Autodesk Inventor part; units mm, degrees
(part 2 of 3)
  spline S259 degree 2 poles (6.7775, 4.9124) (6.7775, 4.5098) (7.1283, 4.0578) (7.4395, 4.0578) knots 0 0 0 1 2 2 2
  spline S260 degree 2 poles (7.4395, 4.0578) (7.6272, 4.0578) (7.9681, 4.2134) (8.099, 4.3344) knots 0 0 0 1 2 2 2
  line L270 (8.099, 4.3344) -> (8.1212, 4.3344)
  line L271 (8.1212, 4.3344) -> (8.1212, 3.9022)
  spline S261 degree 2 poles (8.1212, 3.9022) (8.0644, 3.875) (7.8915, 3.7984) (7.8223, 3.7811) knots 0 0 0 1 2 2 2
  spline S262 degree 2 poles (7.8223, 3.7811) (7.7235, 3.7515) (7.5679, 3.7218) (7.4469, 3.7218) knots 0 0 0 1 2 2 2
  line L272 (10.2677, 3.7737) -> (9.8823, 3.7737)
  line L273 (9.8823, 3.7737) -> (9.8823, 5.0779)
  spline S263 degree 2 poles (9.8823, 5.0779) (9.8823, 5.236) (9.8527, 5.5077) (9.8082, 5.5892) knots 0 0 0 1 2 2 2
  spline S264 degree 2 poles (9.8082, 5.5892) (9.7613, 5.6756) (9.5933, 5.7596) (9.4501, 5.7596) knots 0 0 0 1 2 2 2
  spline S265 degree 2 poles (9.4501, 5.7596) (9.3068, 5.7596) (9.003, 5.6065) (8.8573, 5.483) knots 0 0 0 1 2 2 2
  line L274 (8.8573, 5.483) -> (8.8573, 3.7737)
  line L275 (8.8573, 3.7737) -> (8.472, 3.7737)
  line L276 (8.472, 3.7737) -> (8.472, 6.9576)
  line L277 (8.472, 6.9576) -> (8.8573, 6.9576)
  line L278 (8.8573, 6.9576) -> (8.8573, 5.8065)
  spline S266 degree 2 poles (8.8573, 5.8065) (9.0302, 5.9621) (9.3636, 6.1252) (9.5514, 6.1252) knots 0 0 0 1 2 2 2
  spline S267 degree 2 poles (9.5514, 6.1252) (9.8873, 6.1252) (10.2677, 5.6806) (10.2677, 5.2582) knots 0 0 0 1 2 2 2
  line L279 (10.2677, 5.2582) -> (10.2677, 3.7737)
  line L280 (14.0221, 4.821) -> (13.659, 4.821)
  line L281 (13.659, 4.821) -> (13.659, 3.7737)
  line L282 (13.659, 3.7737) -> (13.2663, 3.7737)
  line L283 (13.2663, 3.7737) -> (13.2663, 4.821)
  line L284 (13.2663, 4.821) -> (11.9201, 4.821)
  line L285 (11.9201, 4.821) -> (11.9201, 5.2508)
  line L286 (11.9201, 5.2508) -> (13.2836, 6.8217)
  line L287 (13.2836, 6.8217) -> (13.659, 6.8217)
  line L288 (13.659, 6.8217) -> (13.659, 5.1495)
  line L289 (13.659, 5.1495) -> (14.0221, 5.1495)
  line L290 (14.0221, 5.1495) -> (14.0221, 4.821)
  line L291 (13.2663, 5.1495) -> (13.2663, 6.3401)
  line L292 (13.2663, 6.3401) -> (12.2412, 5.1495)
  line L293 (12.2412, 5.1495) -> (13.2663, 5.1495)
  line L294 (16.0747, 3.7737) -> (14.5877, 3.7737)
  line L295 (14.5877, 3.7737) -> (14.5877, 4.0849)
  line L296 (14.5877, 4.0849) -> (15.141, 4.0849)
  line L297 (15.141, 4.0849) -> (15.141, 6.1276)
  line L298 (15.141, 6.1276) -> (14.5877, 6.1276)
  line L299 (14.5877, 6.1276) -> (14.5877, 6.4067)
  spline S268 degree 2 poles (14.5877, 6.4067) (14.9014, 6.4067) (15.1978, 6.5846) (15.2176, 6.8316) knots 0 0 0 1 2 2 2
  line L300 (15.2176, 6.8316) -> (15.5337, 6.8316)
  line L301 (15.5337, 6.8316) -> (15.5337, 4.0849)
  line L302 (15.5337, 4.0849) -> (16.0747, 4.0849)
  line L303 (16.0747, 4.0849) -> (16.0747, 3.7737)
  line L304 (17.2899, 3.7737) -> (16.8009, 3.7737)
  line L305 (16.8009, 3.7737) -> (16.8009, 4.3566)
  line L306 (16.8009, 4.3566) -> (17.2899, 4.3566)
  line L307 (17.2899, 4.3566) -> (17.2899, 3.7737)
  spline S269 degree 2 poles (19.8019, 5.2977) (19.8019, 4.4777) (19.3252, 3.7095) (18.8287, 3.7095) knots 0 0 0 1 2 2 2
  spline S270 degree 2 poles (18.8287, 3.7095) (18.3249, 3.7095) (17.8531, 4.4925) (17.8531, 5.2952) knots 0 0 0 1 2 2 2
  spline S271 degree 2 poles (17.8531, 5.2952) (17.8531, 6.1202) (18.3298, 6.8835) (18.8287, 6.8835) knots 0 0 0 1 2 2 2
  spline S272 degree 2 poles (18.8287, 6.8835) (19.3302, 6.8835) (19.8019, 6.0931) (19.8019, 5.2977) knots 0 0 0 1 2 2 2
  spline S273 degree 2 poles (19.2783, 4.369) (19.3376, 4.5197) (19.387, 4.984) (19.387, 5.2977) knots 0 0 0 1 2 2 2
  spline S274 degree 2 poles (19.387, 5.2977) (19.387, 5.6114) (19.3376, 6.0733) (19.2758, 6.2289) knots 0 0 0 1 2 2 2
  spline S275 degree 2 poles (19.2758, 6.2289) (19.2141, 6.3845) (18.9992, 6.5451) (18.8287, 6.5451) knots 0 0 0 1 2 2 2
  spline S276 degree 2 poles (18.8287, 6.5451) (18.6583, 6.5451) (18.4385, 6.3845) (18.3743, 6.224) knots 0 0 0 1 2 2 2
  spline S277 degree 2 poles (18.3743, 6.224) (18.3125, 6.0684) (18.268, 5.5941) (18.268, 5.2952) knots 0 0 0 1 2 2 2
  spline S278 degree 2 poles (18.268, 5.2952) (18.268, 4.9741) (18.3076, 4.5444) (18.3718, 4.3764) knots 0 0 0 1 2 2 2
  spline S279 degree 2 poles (18.3718, 4.3764) (18.4311, 4.2183) (18.6509, 4.0479) (18.8287, 4.0479) knots 0 0 0 1 2 2 2
  spline S280 degree 2 poles (18.8287, 4.0479) (18.9967, 4.0479) (19.2165, 4.2084) (19.2783, 4.369) knots 0 0 0 1 2 2 2
  spline S281 degree 2 poles (22.0892, 5.2977) (22.0892, 4.4777) (21.6124, 3.7095) (21.116, 3.7095) knots 0 0 0 1 2 2 2
  spline S282 degree 2 poles (21.116, 3.7095) (20.6121, 3.7095) (20.1403, 4.4925) (20.1403, 5.2952) knots 0 0 0 1 2 2 2
  spline S283 degree 2 poles (20.1403, 5.2952) (20.1403, 6.1202) (20.617, 6.8835) (21.116, 6.8835) knots 0 0 0 1 2 2 2
  spline S284 degree 2 poles (21.116, 6.8835) (21.6174, 6.8835) (22.0892, 6.0931) (22.0892, 5.2977) knots 0 0 0 1 2 2 2
  spline S285 degree 2 poles (21.5655, 4.369) (21.6248, 4.5197) (21.6742, 4.984) (21.6742, 5.2977) knots 0 0 0 1 2 2 2
  spline S286 degree 2 poles (21.6742, 5.2977) (21.6742, 5.6114) (21.6248, 6.0733) (21.563, 6.2289) knots 0 0 0 1 2 2 2
  spline S287 degree 2 poles (21.563, 6.2289) (21.5013, 6.3845) (21.2864, 6.5451) (21.116, 6.5451) knots 0 0 0 1 2 2 2
  spline S288 degree 2 poles (21.116, 6.5451) (20.9455, 6.5451) (20.7257, 6.3845) (20.6615, 6.224) knots 0 0 0 1 2 2 2
  spline S289 degree 2 poles (20.6615, 6.224) (20.5997, 6.0684) (20.5553, 5.5941) (20.5553, 5.2952) knots 0 0 0 1 2 2 2
  spline S290 degree 2 poles (20.5553, 5.2952) (20.5553, 4.9741) (20.5948, 4.5444) (20.659, 4.3764) knots 0 0 0 1 2 2 2
  spline S291 degree 2 poles (20.659, 4.3764) (20.7183, 4.2183) (20.9381, 4.0479) (21.116, 4.0479) knots 0 0 0 1 2 2 2
  spline S292 degree 2 poles (21.116, 4.0479) (21.2839, 4.0479) (21.5038, 4.2084) (21.5655, 4.369) knots 0 0 0 1 2 2 2
  spline S293 degree 2 poles (23.3019, 6.5327) (23.1908, 6.5327) (22.971, 6.4784) (22.8647, 6.4364) knots 0 0 0 1 2 2 2
  spline S294 degree 2 poles (22.8647, 6.4364) (22.7659, 6.3944) (22.6202, 6.3055) (22.5634, 6.266) knots 0 0 0 1 2 2 2
  line L308 (22.5634, 6.266) -> (22.5387, 6.266)
  line L309 (22.5387, 6.266) -> (22.5387, 6.6982)
  spline S295 degree 2 poles (22.5387, 6.6982) (22.6721, 6.7698) (23.129, 6.8859) (23.334, 6.8859) knots 0 0 0 1 2 2 2
  spline S296 degree 2 poles (23.334, 6.8859) (23.5415, 6.8859) (23.8503, 6.8019) (23.9763, 6.713) knots 0 0 0 1 2 2 2
  spline S297 degree 2 poles (23.9763, 6.713) (24.1096, 6.6167) (24.248, 6.3376) (24.248, 6.1499) knots 0 0 0 1 2 2 2
  spline S298 degree 2 poles (24.248, 6.1499) (24.248, 5.8979) (23.917, 5.5175) (23.6848, 5.4681) knots 0 0 0 1 2 2 2
  line L310 (23.6848, 5.4681) -> (23.6848, 5.4385)
  spline S299 degree 2 poles (23.6848, 5.4385) (23.7811, 5.4187) (24.001, 5.3298) (24.0948, 5.2409) knots 0 0 0 1 2 2 2
  spline S300 degree 2 poles (24.0948, 5.2409) (24.1887, 5.1544) (24.3072, 4.8778) (24.3072, 4.6777) knots 0 0 0 1 2 2 2
  spline S301 degree 2 poles (24.3072, 4.6777) (24.3072, 4.4727) (24.1664, 4.1245) (24.038, 3.9911) knots 0 0 0 1 2 2 2
  spline S302 degree 2 poles (24.038, 3.9911) (23.9046, 3.8527) (23.5267, 3.7095) (23.2871, 3.7095) knots 0 0 0 1 2 2 2
  spline S303 degree 2 poles (23.2871, 3.7095) (23.0574, 3.7095) (22.6079, 3.8206) (22.4547, 3.8972) knots 0 0 0 1 2 2 2
  line L311 (22.4547, 3.8972) -> (22.4547, 4.3295)
  line L312 (22.4547, 4.3295) -> (22.4844, 4.3295)
  spline S304 degree 2 poles (22.4844, 4.3295) (22.6128, 4.2356) (23.0475, 4.0627) (23.2624, 4.0627) knots 0 0 0 1 2 2 2
  spline S305 degree 2 poles (23.2624, 4.0627) (23.3884, 4.0627) (23.6403, 4.1417) (23.7243, 4.2331) knots 0 0 0 1 2 2 2
  spline S306 degree 2 poles (23.7243, 4.2331) (23.8058, 4.3245) (23.8923, 4.5419) (23.8923, 4.7074) knots 0 0 0 1 2 2 2
  spline S307 degree 2 poles (23.8923, 4.7074) (23.8923, 4.8729) (23.7959, 5.0878) (23.7095, 5.1495) knots 0 0 0 1 2 2 2
  spline S308 degree 2 poles (23.7095, 5.1495) (23.623, 5.2113) (23.3884, 5.2582) (23.2501, 5.2582) knots 0 0 0 1 2 2 2
  line L313 (23.2501, 5.2582) -> (23.0772, 5.2582)
  line L314 (23.0772, 5.2582) -> (23.0772, 5.5966)
  line L315 (23.0772, 5.5966) -> (23.213, 5.5966)
  spline S309 degree 2 poles (23.213, 5.5966) (23.4872, 5.5966) (23.833, 5.8584) (23.833, 6.1079) knots 0 0 0 1 2 2 2
  spline S310 degree 2 poles (23.833, 6.1079) (23.833, 6.224) (23.7441, 6.3895) (23.6724, 6.4389) knots 0 0 0 1 2 2 2
  spline S311 degree 2 poles (23.6724, 6.4389) (23.5959, 6.4907) (23.4081, 6.5327) (23.3019, 6.5327) knots 0 0 0 1 2 2 2
  line L316 (27.9085, 3.7737) -> (27.4367, 3.7737)
  line L317 (27.4367, 3.7737) -> (26.881, 4.6333)
  line L318 (26.881, 4.6333) -> (26.3104, 3.7737)
  line L319 (26.3104, 3.7737) -> (25.8732, 3.7737)
  line L320 (25.8732, 3.7737) -> (26.6661, 4.9074)
  line L321 (26.6661, 4.9074) -> (25.8806, 6.0609)
  line L322 (25.8806, 6.0609) -> (26.3524, 6.0609)
  line L323 (26.3524, 6.0609) -> (26.9057, 5.2088)
  line L324 (26.9057, 5.2088) -> (27.4713, 6.0609)
  line L325 (27.4713, 6.0609) -> (27.9085, 6.0609)
  line L326 (27.9085, 6.0609) -> (27.1206, 4.9321)
  line L327 (27.1206, 4.9321) -> (27.9085, 3.7737)
  spline S312 degree 2 poles (30.2822, 6.5327) (30.1711, 6.5327) (29.9512, 6.4784) (29.845, 6.4364) knots 0 0 0 1 2 2 2
  spline S313 degree 2 poles (29.845, 6.4364) (29.7462, 6.3944) (29.6005, 6.3055) (29.5437, 6.266) knots 0 0 0 1 2 2 2
  line L328 (29.5437, 6.266) -> (29.519, 6.266)
  line L329 (29.519, 6.266) -> (29.519, 6.6982)
  spline S314 degree 2 poles (29.519, 6.6982) (29.6523, 6.7698) (30.1093, 6.8859) (30.3143, 6.8859) knots 0 0 0 1 2 2 2
  spline S315 degree 2 poles (30.3143, 6.8859) (30.5218, 6.8859) (30.8305, 6.8019) (30.9565, 6.713) knots 0 0 0 1 2 2 2
  spline S316 degree 2 poles (30.9565, 6.713) (31.0899, 6.6167) (31.2282, 6.3376) (31.2282, 6.1499) knots 0 0 0 1 2 2 2
  spline S317 degree 2 poles (31.2282, 6.1499) (31.2282, 5.8979) (30.8972, 5.5175) (30.6651, 5.4681) knots 0 0 0 1 2 2 2
  line L330 (30.6651, 5.4681) -> (30.6651, 5.4385)
  spline S318 degree 2 poles (30.6651, 5.4385) (30.7614, 5.4187) (30.9812, 5.3298) (31.0751, 5.2409) knots 0 0 0 1 2 2 2
  spline S319 degree 2 poles (31.0751, 5.2409) (31.1689, 5.1544) (31.2875, 4.8778) (31.2875, 4.6777) knots 0 0 0 1 2 2 2
  spline S320 degree 2 poles (31.2875, 4.6777) (31.2875, 4.4727) (31.1467, 4.1245) (31.0183, 3.9911) knots 0 0 0 1 2 2 2
  spline S321 degree 2 poles (31.0183, 3.9911) (30.8849, 3.8527) (30.507, 3.7095) (30.2674, 3.7095) knots 0 0 0 1 2 2 2
  spline S322 degree 2 poles (30.2674, 3.7095) (30.0377, 3.7095) (29.5881, 3.8206) (29.435, 3.8972) knots 0 0 0 1 2 2 2
  line L331 (29.435, 3.8972) -> (29.435, 4.3295)
  line L332 (29.435, 4.3295) -> (29.4646, 4.3295)
  spline S323 degree 2 poles (29.4646, 4.3295) (29.5931, 4.2356) (30.0278, 4.0627) (30.2427, 4.0627) knots 0 0 0 1 2 2 2
  spline S324 degree 2 poles (30.2427, 4.0627) (30.3687, 4.0627) (30.6206, 4.1417) (30.7046, 4.2331) knots 0 0 0 1 2 2 2
  spline S325 degree 2 poles (30.7046, 4.2331) (30.7861, 4.3245) (30.8725, 4.5419) (30.8725, 4.7074) knots 0 0 0 1 2 2 2
  spline S326 degree 2 poles (30.8725, 4.7074) (30.8725, 4.8729) (30.7762, 5.0878) (30.6898, 5.1495) knots 0 0 0 1 2 2 2
  spline S327 degree 2 poles (30.6898, 5.1495) (30.6033, 5.2113) (30.3687, 5.2582) (30.2303, 5.2582) knots 0 0 0 1 2 2 2
  line L333 (30.2303, 5.2582) -> (30.0574, 5.2582)
  line L334 (30.0574, 5.2582) -> (30.0574, 5.5966)
  line L335 (30.0574, 5.5966) -> (30.1933, 5.5966)
  spline S328 degree 2 poles (30.1933, 5.5966) (30.4675, 5.5966) (30.8133, 5.8584) (30.8133, 6.1079) knots 0 0 0 1 2 2 2
  spline S329 degree 2 poles (30.8133, 6.1079) (30.8133, 6.224) (30.7243, 6.3895) (30.6527, 6.4389) knots 0 0 0 1 2 2 2
  spline S330 degree 2 poles (30.6527, 6.4389) (30.5761, 6.4907) (30.3884, 6.5327) (30.2822, 6.5327) knots 0 0 0 1 2 2 2
  line L336 (33.7081, 4.821) -> (33.345, 4.821)
  line L337 (33.345, 4.821) -> (33.345, 3.7737)
  line L338 (33.345, 3.7737) -> (32.9523, 3.7737)
  line L339 (32.9523, 3.7737) -> (32.9523, 4.821)
  line L340 (32.9523, 4.821) -> (31.6061, 4.821)
  line L341 (31.6061, 4.821) -> (31.6061, 5.2508)
  line L342 (31.6061, 5.2508) -> (32.9696, 6.8217)
  line L343 (32.9696, 6.8217) -> (33.345, 6.8217)
  line L344 (33.345, 6.8217) -> (33.345, 5.1495)
  line L345 (33.345, 5.1495) -> (33.7081, 5.1495)
  line L346 (33.7081, 5.1495) -> (33.7081, 4.821)
  line L347 (32.9523, 5.1495) -> (32.9523, 6.3401)
  line L348 (32.9523, 6.3401) -> (31.9272, 5.1495)
  line L349 (31.9272, 5.1495) -> (32.9523, 5.1495)
  line L350 (34.6887, 3.7737) -> (34.1996, 3.7737)
  line L351 (34.1996, 3.7737) -> (34.1996, 4.3566)
  line L352 (34.1996, 4.3566) -> (34.6887, 4.3566)
  line L353 (34.6887, 4.3566) -> (34.6887, 3.7737)
  spline S331 degree 2 poles (36.1263, 6.5327) (36.0151, 6.5327) (35.7953, 6.4784) (35.6891, 6.4364) knots 0 0 0 1 2 2 2
  spline S332 degree 2 poles (35.6891, 6.4364) (35.5903, 6.3944) (35.4445, 6.3055) (35.3877, 6.266) knots 0 0 0 1 2 2 2
  line L354 (35.3877, 6.266) -> (35.363, 6.266)
  line L355 (35.363, 6.266) -> (35.363, 6.6982)
  spline S333 degree 2 poles (35.363, 6.6982) (35.4964, 6.7698) (35.9534, 6.8859) (36.1584, 6.8859) knots 0 0 0 1 2 2 2
  spline S334 degree 2 poles (36.1584, 6.8859) (36.3659, 6.8859) (36.6746, 6.8019) (36.8006, 6.713) knots 0 0 0 1 2 2 2
  spline S335 degree 2 poles (36.8006, 6.713) (36.934, 6.6167) (37.0723, 6.3376) (37.0723, 6.1499) knots 0 0 0 1 2 2 2
  spline S336 degree 2 poles (37.0723, 6.1499) (37.0723, 5.8979) (36.7413, 5.5175) (36.5091, 5.4681) knots 0 0 0 1 2 2 2
  line L356 (36.5091, 5.4681) -> (36.5091, 5.4385)
  spline S337 degree 2 poles (36.5091, 5.4385) (36.6054, 5.4187) (36.8253, 5.3298) (36.9191, 5.2409) knots 0 0 0 1 2 2 2
  spline S338 degree 2 poles (36.9191, 5.2409) (37.013, 5.1544) (37.1316, 4.8778) (37.1316, 4.6777) knots 0 0 0 1 2 2 2
  spline S339 degree 2 poles (37.1316, 4.6777) (37.1316, 4.4727) (36.9908, 4.1245) (36.8623, 3.9911) knots 0 0 0 1 2 2 2
  spline S340 degree 2 poles (36.8623, 3.9911) (36.7289, 3.8527) (36.351, 3.7095) (36.1114, 3.7095) knots 0 0 0 1 2 2 2
  spline S341 degree 2 poles (36.1114, 3.7095) (35.8817, 3.7095) (35.4322, 3.8206) (35.279, 3.8972) knots 0 0 0 1 2 2 2
  line L357 (35.279, 3.8972) -> (35.279, 4.3295)
  line L358 (35.279, 4.3295) -> (35.3087, 4.3295)
  spline S342 degree 2 poles (35.3087, 4.3295) (35.4371, 4.2356) (35.8719, 4.0627) (36.0867, 4.0627) knots 0 0 0 1 2 2 2
  spline S343 degree 2 poles (36.0867, 4.0627) (36.2127, 4.0627) (36.4647, 4.1417) (36.5486, 4.2331) knots 0 0 0 1 2 2 2
  spline S344 degree 2 poles (36.5486, 4.2331) (36.6301, 4.3245) (36.7166, 4.5419) (36.7166, 4.7074) knots 0 0 0 1 2 2 2
  spline S345 degree 2 poles (36.7166, 4.7074) (36.7166, 4.8729) (36.6203, 5.0878) (36.5338, 5.1495) knots 0 0 0 1 2 2 2
  spline S346 degree 2 poles (36.5338, 5.1495) (36.4474, 5.2113) (36.2127, 5.2582) (36.0744, 5.2582) knots 0 0 0 1 2 2 2
  line L359 (36.0744, 5.2582) -> (35.9015, 5.2582)
  line L360 (35.9015, 5.2582) -> (35.9015, 5.5966)
  line L361 (35.9015, 5.5966) -> (36.0373, 5.5966)
  spline S347 degree 2 poles (36.0373, 5.5966) (36.3115, 5.5966) (36.6573, 5.8584) (36.6573, 6.1079) knots 0 0 0 1 2 2 2
  spline S348 degree 2 poles (36.6573, 6.1079) (36.6573, 6.224) (36.5684, 6.3895) (36.4968, 6.4389) knots 0 0 0 1 2 2 2
  spline S349 degree 2 poles (36.4968, 6.4389) (36.4202, 6.4907) (36.2325, 6.5327) (36.1263, 6.5327) knots 0 0 0 1 2 2 2
  spline S350 degree 2 poles (39.4386, 4.742) (39.4386, 4.5221) (39.2978, 4.1467) (39.1693, 4.0084) knots 0 0 0 1 2 2 2
  spline S351 degree 2 poles (39.1693, 4.0084) (39.0409, 3.87) (38.658, 3.7095) (38.4209, 3.7095) knots 0 0 0 1 2 2 2
  spline S352 degree 2 poles (38.4209, 3.7095) (38.2035, 3.7095) (37.7787, 3.8058) (37.6231, 3.8824) knots 0 0 0 1 2 2 2
  line L362 (37.6231, 3.8824) -> (37.6231, 4.3146)
  line L363 (37.6231, 4.3146) -> (37.6527, 4.3146)
  spline S353 degree 2 poles (37.6527, 4.3146) (37.6997, 4.2801) (37.875, 4.1911) (37.9812, 4.1516) knots 0 0 0 1 2 2 2
  spline S354 degree 2 poles (37.9812, 4.1516) (38.1023, 4.1096) (38.3023, 4.0627) (38.4283, 4.0627) knots 0 0 0 1 2 2 2
  spline S355 degree 2 poles (38.4283, 4.0627) (38.5518, 4.0627) (38.784, 4.1516) (38.868, 4.248) knots 0 0 0 1 2 2 2
  spline S356 degree 2 poles (38.868, 4.248) (38.9446, 4.3393) (39.0236, 4.5814) (39.0236, 4.7444) knots 0 0 0 1 2 2 2
  spline S357 degree 2 poles (39.0236, 4.7444) (39.0236, 4.9074) (38.9347, 5.1149) (38.8507, 5.1841) knots 0 0 0 1 2 2 2
  spline S358 degree 2 poles (38.8507, 5.1841) (38.7642, 5.2607) (38.5074, 5.3249) (38.3517, 5.3249) knots 0 0 0 1 2 2 2
  spline S359 degree 2 poles (38.3517, 5.3249) (38.1838, 5.3249) (37.8503, 5.273) (37.7491, 5.2508) knots 0 0 0 1 2 2 2
  line L364 (37.7491, 5.2508) -> (37.7491, 6.8217)
  line L365 (37.7491, 6.8217) -> (39.4213, 6.8217)
  line L366 (39.4213, 6.8217) -> (39.4213, 6.4636)
  line L367 (39.4213, 6.4636) -> (38.1418, 6.4636)
  line L368 (38.1418, 6.4636) -> (38.1418, 5.6509)
  spline S360 degree 2 poles (38.1418, 5.6509) (38.2159, 5.6608) (38.3592, 5.6682) (38.4184, 5.6682) knots 0 0 0 1 2 2 2
  spline S361 degree 2 poles (38.4184, 5.6682) (38.6531, 5.6682) (38.9767, 5.5916) (39.1249, 5.478) knots 0 0 0 1 2 2 2
  spline S362 degree 2 poles (39.1249, 5.478) (39.2755, 5.3644) (39.4386, 5.0186) (39.4386, 4.742) knots 0 0 0 1 2 2 2
  spline S363 degree 2 poles (39.7942, 5.8312) (39.7942, 6.0659) (39.9474, 6.4561) (40.0808, 6.5969) knots 0 0 0 1 2 2 2
  spline S364 degree 2 poles (40.0808, 6.5969) (40.2067, 6.7328) (40.5748, 6.8835) (40.7625, 6.8835) knots 0 0 0 1 2 2 2
  spline S365 degree 2 poles (40.7625, 6.8835) (40.9724, 6.8835) (41.3133, 6.7427) (41.4393, 6.6093) knots 0 0 0 1 2 2 2
  spline S366 degree 2 poles (41.4393, 6.6093) (41.5973, 6.4413) (41.7702, 5.8979) (41.7702, 5.4805) knots 0 0 0 1 2 2 2
  spline S367 degree 2 poles (41.7702, 5.4805) (41.7702, 5.1026) (41.5998, 4.4258) (41.4343, 4.201) knots 0 0 0 1 2 2 2
  spline S368 degree 2 poles (41.4343, 4.201) (41.259, 3.9639) (40.765, 3.7144) (40.4043, 3.7144) knots 0 0 0 1 2 2 2
  spline S369 degree 2 poles (40.4043, 3.7144) (40.3228, 3.7144) (40.1376, 3.7317) (40.0585, 3.7564) knots 0 0 0 1 2 2 2
  line L369 (40.0585, 3.7564) -> (40.0585, 4.1492)
  line L370 (40.0585, 4.1492) -> (40.0783, 4.1492)
  spline S370 degree 2 poles (40.0783, 4.1492) (40.1302, 4.1195) (40.3475, 4.0676) (40.4587, 4.0676) knots 0 0 0 1 2 2 2
  spline S371 degree 2 poles (40.4587, 4.0676) (40.8588, 4.0676) (41.3158, 4.5962) (41.3479, 5.0853) knots 0 0 0 1 2 2 2
  spline S372 degree 2 poles (41.3479, 5.0853) (41.1849, 4.9741) (40.8885, 4.8729) (40.7131, 4.8729) knots 0 0 0 1 2 2 2
  spline S373 degree 2 poles (40.7131, 4.8729) (40.5451, 4.8729) (40.266, 4.947) (40.1252, 5.0532) knots 0 0 0 1 2 2 2
  spline S374 degree 2 poles (40.1252, 5.0532) (39.9622, 5.1791) (39.7942, 5.562) (39.7942, 5.8312) knots 0 0 0 1 2 2 2
  spline S375 degree 2 poles (41.3578, 5.5719) (41.3578, 5.8806) (41.2441, 6.2709) (41.1429, 6.3771) knots 0 0 0 1 2 2 2
  spline S376 degree 2 poles (41.1429, 6.3771) (41.0539, 6.4759) (40.8687, 6.55) (40.76, 6.55) knots 0 0 0 1 2 2 2
  spline S377 degree 2 poles (40.76, 6.55) (40.5081, 6.55) (40.2092, 6.1894) (40.2092, 5.8485) knots 0 0 0 1 2 2 2
  spline S378 degree 2 poles (40.2092, 5.8485) (40.2092, 5.6559) (40.308, 5.4064) (40.4167, 5.3175) knots 0 0 0 1 2 2 2
  spline S379 degree 2 poles (40.4167, 5.3175) (40.4957, 5.2532) (40.6909, 5.2113) (40.8045, 5.2113) knots 0 0 0 1 2 2 2
  spline S380 degree 2 poles (40.8045, 5.2113) (40.9354, 5.2113) (41.2367, 5.3026) (41.3503, 5.3792) knots 0 0 0 1 2 2 2
  spline S381 degree 2 poles (41.3503, 5.3792) (41.3528, 5.4089) (41.3578, 5.5101) (41.3578, 5.5719) knots 0 0 0 1 2 2 2
  spline S382 degree 2 poles (45.4111, 4.9173) (45.4111, 4.3393) (44.8553, 3.7095) (44.3909, 3.7095) knots 0 0 0 1 2 2 2
  spline S383 degree 2 poles (44.3909, 3.7095) (43.9142, 3.7095) (43.3684, 4.3591) (43.3684, 4.9173) knots 0 0 0 1 2 2 2
  spline S384 degree 2 poles (43.3684, 4.9173) (43.3684, 5.4904) (43.9315, 6.1252) (44.3909, 6.1252) knots 0 0 0 1 2 2 2
  spline S385 degree 2 poles (44.3909, 6.1252) (44.8553, 6.1252) (45.4111, 5.4928) (45.4111, 4.9173) knots 0 0 0 1 2 2 2
  spline S386 degree 2 poles (45.0134, 4.9173) (45.0134, 5.3619) (44.6898, 5.7942) (44.3909, 5.7942) knots 0 0 0 1 2 2 2
  spline S387 degree 2 poles (44.3909, 5.7942) (44.0921, 5.7942) (43.766, 5.3619) (43.766, 4.9173) knots 0 0 0 1 2 2 2
  spline S388 degree 2 poles (43.766, 4.9173) (43.766, 4.4851) (44.0921, 4.0405) (44.3909, 4.0405) knots 0 0 0 1 2 2 2
  spline S389 degree 2 poles (44.3909, 4.0405) (44.6873, 4.0405) (45.0134, 4.4777) (45.0134, 4.9173) knots 0 0 0 1 2 2 2
  line L371 (47.0092, 6.5871) -> (46.9894, 6.5871)
  spline S390 degree 2 poles (46.9894, 6.5871) (46.9375, 6.6068) (46.7449, 6.6414) (46.6683, 6.6414) knots 0 0 0 1 2 2 2
  spline S391 degree 2 poles (46.6683, 6.6414) (46.4262, 6.6414) (46.2187, 6.424) (46.2187, 6.1375) knots 0 0 0 1 2 2 2
  line L372 (46.2187, 6.1375) -> (46.2187, 6.0609)
  line L373 (46.2187, 6.0609) -> (46.856, 6.0609)
  line L374 (46.856, 6.0609) -> (46.856, 5.7423)
  line L375 (46.856, 5.7423) -> (46.2311, 5.7423)
  line L376 (46.2311, 5.7423) -> (46.2311, 3.7737)
  line L377 (46.2311, 3.7737) -> (45.8458, 3.7737)
  line L378 (45.8458, 3.7737) -> (45.8458, 5.7423)
  line L379 (45.8458, 5.7423) -> (45.5864, 5.7423)
  line L380 (45.5864, 5.7423) -> (45.5864, 6.0609)
  line L381 (45.5864, 6.0609) -> (45.8458, 6.0609)
  line L382 (45.8458, 6.0609) -> (45.8458, 6.1375)
  spline S392 degree 2 poles (45.8458, 6.1375) (45.8458, 6.5475) (46.2434, 6.9773) (46.614, 6.9773) knots 0 0 0 1 2 2 2
  spline S393 degree 2 poles (46.614, 6.9773) (46.7202, 6.9773) (46.9252, 6.9551) (47.0092, 6.9403) knots 0 0 0 1 2 2 2
  line L383 (47.0092, 6.9403) -> (47.0092, 6.5871)
  line L384 (48.343, 6.5871) -> (48.3232, 6.5871)
  spline S394 degree 2 poles (48.3232, 6.5871) (48.2713, 6.6068) (48.0787, 6.6414) (48.0021, 6.6414) knots 0 0 0 1 2 2 2
  spline S395 degree 2 poles (48.0021, 6.6414) (47.76, 6.6414) (47.5526, 6.424) (47.5526, 6.1375) knots 0 0 0 1 2 2 2
  line L385 (47.5526, 6.1375) -> (47.5526, 6.0609)
  line L386 (47.5526, 6.0609) -> (48.1898, 6.0609)
  line L387 (48.1898, 6.0609) -> (48.1898, 5.7423)
  line L388 (48.1898, 5.7423) -> (47.5649, 5.7423)
  line L389 (47.5649, 5.7423) -> (47.5649, 3.7737)
  line L390 (47.5649, 3.7737) -> (47.1796, 3.7737)
  line L391 (47.1796, 3.7737) -> (47.1796, 5.7423)
  line L392 (47.1796, 5.7423) -> (46.9202, 5.7423)
  line L393 (46.9202, 5.7423) -> (46.9202, 6.0609)
  line L394 (46.9202, 6.0609) -> (47.1796, 6.0609)
  line L395 (47.1796, 6.0609) -> (47.1796, 6.1375)
  spline S396 degree 2 poles (47.1796, 6.1375) (47.1796, 6.5475) (47.5773, 6.9773) (47.9478, 6.9773) knots 0 0 0 1 2 2 2
  spline S397 degree 2 poles (47.9478, 6.9773) (48.054, 6.9773) (48.259, 6.9551) (48.343, 6.9403) knots 0 0 0 1 2 2 2
  line L396 (48.343, 6.9403) -> (48.343, 6.5871)
  spline S398 degree 2 poles (49.0914, 3.7194) (48.8617, 3.7194) (48.464, 3.8429) (48.3331, 3.912) knots 0 0 0 1 2 2 2
  line L397 (48.3331, 3.912) -> (48.3331, 4.3443)
  line L398 (48.3331, 4.3443) -> (48.3528, 4.3443)
  spline S399 degree 2 poles (48.3528, 4.3443) (48.4022, 4.3048) (48.5356, 4.2109) (48.6468, 4.159) knots 0 0 0 1 2 2 2
  spline S400 degree 2 poles (48.6468, 4.159) (48.7431, 4.1121) (48.9802, 4.0429) (49.1062, 4.0429) knots 0 0 0 1 2 2 2
  spline S401 degree 2 poles (49.1062, 4.0429) (49.1976, 4.0429) (49.4075, 4.0849) (49.4569, 4.1195) knots 0 0 0 1 2 2 2
  spline S402 degree 2 poles (49.4569, 4.1195) (49.5286, 4.1664) (49.5928, 4.2727) (49.5928, 4.3813) knots 0 0 0 1 2 2 2
  spline S403 degree 2 poles (49.5928, 4.3813) (49.5928, 4.5172) (49.4446, 4.658) (49.2544, 4.7049) knots 0 0 0 1 2 2 2
  spline S404 degree 2 poles (49.2544, 4.7049) (49.1803, 4.7222) (48.9432, 4.7716) (48.8419, 4.7988) knots 0 0 0 1 2 2 2
  spline S405 degree 2 poles (48.8419, 4.7988) (48.5801, 4.8753) (48.343, 5.1915) (48.343, 5.4163) knots 0 0 0 1 2 2 2
  spline S406 degree 2 poles (48.343, 5.4163) (48.343, 5.7275) (48.8098, 6.1153) (49.1951, 6.1153) knots 0 0 0 1 2 2 2
  spline S407 degree 2 poles (49.1951, 6.1153) (49.3853, 6.1153) (49.7706, 6.0214) (49.9015, 5.9498) knots 0 0 0 1 2 2 2
  line L399 (49.9015, 5.9498) -> (49.9015, 5.5373)
  line L400 (49.9015, 5.5373) -> (49.8818, 5.5373)
  spline S408 degree 2 poles (49.8818, 5.5373) (49.7336, 5.6559) (49.373, 5.7917) (49.1877, 5.7917) knots 0 0 0 1 2 2 2
  spline S409 degree 2 poles (49.1877, 5.7917) (48.9975, 5.7917) (48.7357, 5.6312) (48.7357, 5.4706) knots 0 0 0 1 2 2 2
  spline S410 degree 2 poles (48.7357, 5.4706) (48.7357, 5.3249) (48.8913, 5.1841) (49.0642, 5.1396) knots 0 0 0 1 2 2 2
  spline S411 degree 2 poles (49.0642, 5.1396) (49.1482, 5.1174) (49.3606, 5.0729) (49.4767, 5.0458) knots 0 0 0 1 2 2 2
  spline S412 degree 2 poles (49.4767, 5.0458) (49.7286, 4.9815) (49.9855, 4.6876) (49.9855, 4.4332) knots 0 0 0 1 2 2 2
  spline S413 degree 2 poles (49.9855, 4.4332) (49.9855, 4.285) (49.8694, 4.0232) (49.7558, 3.9269) knots 0 0 0 1 2 2 2
  spline S414 degree 2 poles (49.7558, 3.9269) (49.6348, 3.8256) (49.326, 3.7194) (49.0914, 3.7194) knots 0 0 0 1 2 2 2
  spline S415 degree 2 poles (51.3366, 3.7218) (50.7883, 3.7218) (50.1856, 4.3369) (50.1856, 4.905) knots 0 0 0 1 2 2 2
  spline S416 degree 2 poles (50.1856, 4.905) (50.1856, 5.4632) (50.771, 6.1252) (51.2428, 6.1252) knots 0 0 0 1 2 2 2
  spline S417 degree 2 poles (51.2428, 6.1252) (51.4552, 6.1252) (51.7837, 6.0017) (51.9047, 5.8708) knots 0 0 0 1 2 2 2
  spline S418 degree 2 poles (51.9047, 5.8708) (52.0282, 5.7398) (52.1591, 5.3619) (52.1591, 5.0878) knots 0 0 0 1 2 2 2
  line L401 (52.1591, 5.0878) -> (52.1591, 4.8778)
  line L402 (52.1591, 4.8778) -> (50.5759, 4.8778)
  spline S419 degree 2 poles (50.5759, 4.8778) (50.5759, 4.4801) (50.976, 4.0578) (51.3317, 4.0578) knots 0 0 0 1 2 2 2
  spline S420 degree 2 poles (51.3317, 4.0578) (51.4577, 4.0578) (51.7022, 4.1146) (51.801, 4.159) knots 0 0 0 1 2 2 2
  spline S421 degree 2 poles (51.801, 4.159) (51.9047, 4.2084) (52.048, 4.2949) (52.0949, 4.3344) knots 0 0 0 1 2 2 2
  line L403 (52.0949, 4.3344) -> (52.1171, 4.3344)
  line L404 (52.1171, 4.3344) -> (52.1171, 3.9145)
  spline S422 degree 2 poles (52.1171, 3.9145) (52.0505, 3.8873) (51.8479, 3.8083) (51.7689, 3.7861) knots 0 0 0 1 2 2 2
  spline S423 degree 2 poles (51.7689, 3.7861) (51.6577, 3.7539) (51.4749, 3.7218) (51.3366, 3.7218) knots 0 0 0 1 2 2 2
  spline S424 degree 2 poles (51.7837, 5.1717) (51.7788, 5.3273) (51.7145, 5.5546) (51.6528, 5.6312) knots 0 0 0 1 2 2 2
  spline S425 degree 2 poles (51.6528, 5.6312) (51.5861, 5.7176) (51.3761, 5.809) (51.2205, 5.809) knots 0 0 0 1 2 2 2
  spline S426 degree 2 poles (51.2205, 5.809) (51.0674, 5.809) (50.8525, 5.7176) (50.7636, 5.6287) knots 0 0 0 1 2 2 2
  spline S427 degree 2 poles (50.7636, 5.6287) (50.6771, 5.5373) (50.5882, 5.3175) (50.5759, 5.1717) knots 0 0 0 1 2 2 2
  line L405 (50.5759, 5.1717) -> (51.7837, 5.1717)
  spline S428 degree 2 poles (53.241, 3.7292) (52.9273, 3.7292) (52.5741, 4.0874) (52.5741, 4.4752) knots 0 0 0 1 2 2 2
  line L406 (52.5741, 4.4752) -> (52.5741, 5.7423)
  line L407 (52.5741, 5.7423) -> (52.3147, 5.7423)
  line L408 (52.3147, 5.7423) -> (52.3147, 6.0609)
  line L409 (52.3147, 6.0609) -> (52.5741, 6.0609)
  line L410 (52.5741, 6.0609) -> (52.5741, 6.718)
  line L411 (52.5741, 6.718) -> (52.9594, 6.718)
  line L412 (52.9594, 6.718) -> (52.9594, 6.0609)
  line L413 (52.9594, 6.0609) -> (53.6683, 6.0609)
  line L414 (53.6683, 6.0609) -> (53.6683, 5.7423)
  line L415 (53.6683, 5.7423) -> (52.9594, 5.7423)
  line L416 (52.9594, 5.7423) -> (52.9594, 4.653)
  spline S429 degree 2 poles (52.9594, 4.653) (52.9594, 4.4801) (52.9718, 4.2899) (53.0138, 4.2084) knots 0 0 0 1 2 2 2
  spline S430 degree 2 poles (53.0138, 4.2084) (53.0483, 4.1368) (53.204, 4.0652) (53.3373, 4.0652) knots 0 0 0 1 2 2 2
  spline S431 degree 2 poles (53.3373, 4.0652) (53.4312, 4.0652) (53.6066, 4.122) (53.6461, 4.1393) knots 0 0 0 1 2 2 2
  line L417 (53.6461, 4.1393) -> (53.6683, 4.1393)
  line L418 (53.6683, 4.1393) -> (53.6683, 3.7935)
  spline S432 degree 2 poles (53.6683, 3.7935) (53.5596, 3.7638) (53.3373, 3.7292) (53.241, 3.7292) knots 0 0 0 1 2 2 2
  line L419 (57.0844, 3.7737) -> (55.2047, 3.7737)
  line L420 (55.2047, 3.7737) -> (55.2047, 4.206)
  spline S433 degree 2 poles (55.2047, 4.206) (55.4072, 4.3962) (55.7678, 4.7494) (55.9407, 4.9396) knots 0 0 0 1 2 2 2
  spline S434 degree 2 poles (55.9407, 4.9396) (56.289, 5.3224) (56.5434, 5.7818) (56.5434, 6.0264) knots 0 0 0 1 2 2 2
  spline S435 degree 2 poles (56.5434, 6.0264) (56.5434, 6.1548) (56.4644, 6.3475) (56.3927, 6.4092) knots 0 0 0 1 2 2 2
  spline S436 degree 2 poles (56.3927, 6.4092) (56.3211, 6.471) (56.1334, 6.5327) (56.0198, 6.5327) knots 0 0 0 1 2 2 2
  spline S437 degree 2 poles (56.0198, 6.5327) (55.9111, 6.5327) (55.6888, 6.4784) (55.5875, 6.4364) knots 0 0 0 1 2 2 2
  spline S438 degree 2 poles (55.5875, 6.4364) (55.5011, 6.4018) (55.3405, 6.303) (55.2911, 6.2684) knots 0 0 0 1 2 2 2
  line L421 (55.2911, 6.2684) -> (55.2689, 6.2684)
  line L422 (55.2689, 6.2684) -> (55.2689, 6.7031)
  spline S439 degree 2 poles (55.2689, 6.7031) (55.3949, 6.7649) (55.8469, 6.8859) (56.0494, 6.8859) knots 0 0 0 1 2 2 2
  spline S440 degree 2 poles (56.0494, 6.8859) (56.4767, 6.8859) (56.9584, 6.4339) (56.9584, 6.0486) knots 0 0 0 1 2 2 2
  spline S441 degree 2 poles (56.9584, 6.0486) (56.9584, 5.8683) (56.8744, 5.5669) (56.8003, 5.4385) knots 0 0 0 1 2 2 2
  spline S442 degree 2 poles (56.8003, 5.4385) (56.7262, 5.3051) (56.5113, 5.0433) (56.3927, 4.9173) knots 0 0 0 1 2 2 2
  spline S443 degree 2 poles (56.3927, 4.9173) (56.2001, 4.7074) (55.7283, 4.2578) (55.5875, 4.1269) knots 0 0 0 1 2 2 2
  line L423 (55.5875, 4.1269) -> (57.0844, 4.1269)
  line L424 (57.0844, 4.1269) -> (57.0844, 3.7737)
  line L425 (58.1465, 3.7737) -> (57.6574, 3.7737)
  line L426 (57.6574, 3.7737) -> (57.6574, 4.3566)
  line L427 (57.6574, 4.3566) -> (58.1465, 4.3566)
  line L428 (58.1465, 4.3566) -> (58.1465, 3.7737)
  line L429 (60.6758, 6.3648) -> (59.3568, 3.7737)
  line L430 (59.3568, 3.7737) -> (58.922, 3.7737)
  line L431 (58.922, 3.7737) -> (60.3151, 6.4636)
  line L432 (60.3151, 6.4636) -> (58.7417, 6.4636)
  line L433 (58.7417, 6.4636) -> (58.7417, 6.8217)
  line L434 (58.7417, 6.8217) -> (60.6758, 6.8217)
  line L435 (60.6758, 6.8217) -> (60.6758, 6.3648)
  spline S444 degree 2 poles (62.8963, 4.742) (62.8963, 4.5221) (62.7555, 4.1467) (62.6271, 4.0084) knots 0 0 0 1 2 2 2
  spline S445 degree 2 poles (62.6271, 4.0084) (62.4986, 3.87) (62.1158, 3.7095) (61.8787, 3.7095) knots 0 0 0 1 2 2 2
  spline S446 degree 2 poles (61.8787, 3.7095) (61.6613, 3.7095) (61.2364, 3.8058) (61.0808, 3.8824) knots 0 0 0 1 2 2 2
  line L436 (61.0808, 3.8824) -> (61.0808, 4.3146)
  line L437 (61.0808, 4.3146) -> (61.1105, 4.3146)
  spline S447 degree 2 poles (61.1105, 4.3146) (61.1574, 4.2801) (61.3328, 4.1911) (61.439, 4.1516) knots 0 0 0 1 2 2 2
  spline S448 degree 2 poles (61.439, 4.1516) (61.56, 4.1096) (61.7601, 4.0627) (61.8861, 4.0627) knots 0 0 0 1 2 2 2
  spline S449 degree 2 poles (61.8861, 4.0627) (62.0096, 4.0627) (62.2417, 4.1516) (62.3257, 4.248) knots 0 0 0 1 2 2 2
  spline S450 degree 2 poles (62.3257, 4.248) (62.4023, 4.3393) (62.4813, 4.5814) (62.4813, 4.7444) knots 0 0 0 1 2 2 2
  spline S451 degree 2 poles (62.4813, 4.7444) (62.4813, 4.9074) (62.3924, 5.1149) (62.3084, 5.1841) knots 0 0 0 1 2 2 2
  spline S452 degree 2 poles (62.3084, 5.1841) (62.222, 5.2607) (61.9651, 5.3249) (61.8095, 5.3249) knots 0 0 0 1 2 2 2
  spline S453 degree 2 poles (61.8095, 5.3249) (61.6415, 5.3249) (61.3081, 5.273) (61.2068, 5.2508) knots 0 0 0 1 2 2 2
  line L438 (61.2068, 5.2508) -> (61.2068, 6.8217)
  line L439 (61.2068, 6.8217) -> (62.879, 6.8217)
  line L440 (62.879, 6.8217) -> (62.879, 6.4636)
  line L441 (62.879, 6.4636) -> (61.5995, 6.4636)
  line L442 (61.5995, 6.4636) -> (61.5995, 5.6509)
  spline S454 degree 2 poles (61.5995, 5.6509) (61.6736, 5.6608) (61.8169, 5.6682) (61.8762, 5.6682) knots 0 0 0 1 2 2 2
  spline S455 degree 2 poles (61.8762, 5.6682) (62.1108, 5.6682) (62.4344, 5.5916) (62.5826, 5.478) knots 0 0 0 1 2 2 2
  spline S456 degree 2 poles (62.5826, 5.478) (62.7333, 5.3644) (62.8963, 5.0186) (62.8963, 4.742) knots 0 0 0 1 2 2 2
  spline S457 degree 2 poles (65.2329, 5.2977) (65.2329, 4.4777) (64.7562, 3.7095) (64.2597, 3.7095) knots 0 0 0 1 2 2 2
  spline S458 degree 2 poles (64.2597, 3.7095) (63.7559, 3.7095) (63.2841, 4.4925) (63.2841, 5.2952) knots 0 0 0 1 2 2 2
  spline S459 degree 2 poles (63.2841, 5.2952) (63.2841, 6.1202) (63.7608, 6.8835) (64.2597, 6.8835) knots 0 0 0 1 2 2 2
  spline S460 degree 2 poles (64.2597, 6.8835) (64.7612, 6.8835) (65.2329, 6.0931) (65.2329, 5.2977) knots 0 0 0 1 2 2 2
  spline S461 degree 2 poles (64.7093, 4.369) (64.7686, 4.5197) (64.818, 4.984) (64.818, 5.2977) knots 0 0 0 1 2 2 2
  spline S462 degree 2 poles (64.818, 5.2977) (64.818, 5.6114) (64.7686, 6.0733) (64.7068, 6.2289) knots 0 0 0 1 2 2 2
  spline S463 degree 2 poles (64.7068, 6.2289) (64.6451, 6.3845) (64.4302, 6.5451) (64.2597, 6.5451) knots 0 0 0 1 2 2 2
  spline S464 degree 2 poles (64.2597, 6.5451) (64.0893, 6.5451) (63.8695, 6.3845) (63.8053, 6.224) knots 0 0 0 1 2 2 2
  spline S465 degree 2 poles (63.8053, 6.224) (63.7435, 6.0684) (63.6991, 5.5941) (63.6991, 5.2952) knots 0 0 0 1 2 2 2
  spline S466 degree 2 poles (63.6991, 5.2952) (63.6991, 4.9741) (63.7386, 4.5444) (63.8028, 4.3764) knots 0 0 0 1 2 2 2
  spline S467 degree 2 poles (63.8028, 4.3764) (63.8621, 4.2183) (64.0819, 4.0479) (64.2597, 4.0479) knots 0 0 0 1 2 2 2
  spline S468 degree 2 poles (64.2597, 4.0479) (64.4277, 4.0479) (64.6475, 4.2084) (64.7093, 4.369) knots 0 0 0 1 2 2 2
  line L443 (68.7651, 3.7737) -> (68.2933, 3.7737)
  line L444 (68.2933, 3.7737) -> (67.7375, 4.6333)
  line L445 (67.7375, 4.6333) -> (67.167, 3.7737)
  line L446 (67.167, 3.7737) -> (66.7298, 3.7737)
  line L447 (66.7298, 3.7737) -> (67.5226, 4.9074)
  line L448 (67.5226, 4.9074) -> (66.7372, 6.0609)
  line L449 (66.7372, 6.0609) -> (67.2089, 6.0609)
  line L450 (67.2089, 6.0609) -> (67.7622, 5.2088)
  line L451 (67.7622, 5.2088) -> (68.3279, 6.0609)
  line L452 (68.3279, 6.0609) -> (68.7651, 6.0609)
  line L453 (68.7651, 6.0609) -> (67.9771, 4.9321)
  line L454 (67.9771, 4.9321) -> (68.7651, 3.7737)
  spline S469 degree 2 poles (72.2428, 4.7617) (72.2428, 4.5271) (72.0872, 4.1294) (71.9563, 3.996) knots 0 0 0 1 2 2 2
  spline S470 degree 2 poles (71.9563, 3.996) (71.8205, 3.8552) (71.4796, 3.7095) (71.2746, 3.7095) knots 0 0 0 1 2 2 2
  spline S471 degree 2 poles (71.2746, 3.7095) (71.0696, 3.7095) (70.7312, 3.8478) (70.6027, 3.9861) knots 0 0 0 1 2 2 2
  spline S472 degree 2 poles (70.6027, 3.9861) (70.4447, 4.1516) (70.2668, 4.7074) (70.2668, 5.1125) knots 0 0 0 1 2 2 2
  spline S473 degree 2 poles (70.2668, 5.1125) (70.2668, 5.5101) (70.4298, 6.1499) (70.6003, 6.387) knots 0 0 0 1 2 2 2
  spline S474 degree 2 poles (70.6003, 6.387) (70.7658, 6.6192) (71.2894, 6.8785) (71.6327, 6.8785) knots 0 0 0 1 2 2 2
  spline S475 degree 2 poles (71.6327, 6.8785) (71.734, 6.8785) (71.9119, 6.8588) (71.9785, 6.8365) knots 0 0 0 1 2 2 2
  line L455 (71.9785, 6.8365) -> (71.9785, 6.4438)
  line L456 (71.9785, 6.4438) -> (71.9613, 6.4438)
  spline S476 degree 2 poles (71.9613, 6.4438) (71.9044, 6.4734) (71.697, 6.5253) (71.5784, 6.5253) knots 0 0 0 1 2 2 2
  spline S477 degree 2 poles (71.5784, 6.5253) (71.198, 6.5253) (70.7312, 6.0115) (70.6867, 5.5077) knots 0 0 0 1 2 2 2
  spline S478 degree 2 poles (70.6867, 5.5077) (70.8325, 5.6089) (71.1387, 5.7201) (71.3215, 5.7201) knots 0 0 0 1 2 2 2
  spline S479 degree 2 poles (71.3215, 5.7201) (71.4994, 5.7201) (71.7661, 5.6485) (71.9119, 5.5398) knots 0 0 0 1 2 2 2
  spline S480 degree 2 poles (71.9119, 5.5398) (72.0798, 5.4138) (72.2428, 5.0235) (72.2428, 4.7617) knots 0 0 0 1 2 2 2
  spline S481 degree 2 poles (71.8279, 4.7444) (71.8279, 4.9321) (71.7291, 5.1866) (71.6204, 5.2755) knots 0 0 0 1 2 2 2
  spline S482 degree 2 poles (71.6204, 5.2755) (71.5389, 5.3397) (71.3363, 5.3817) (71.2301, 5.3817) knots 0 0 0 1 2 2 2
  spline S483 degree 2 poles (71.2301, 5.3817) (71.0869, 5.3817) (70.8176, 5.2952) (70.6867, 5.2137) knots 0 0 0 1 2 2 2
  spline S484 degree 2 poles (70.6867, 5.2137) (70.6843, 5.1693) (70.6793, 5.0853) (70.6793, 5.0211) knots 0 0 0 1 2 2 2
  spline S485 degree 2 poles (70.6793, 5.0211) (70.6793, 4.7049) (70.8028, 4.3171) (70.8967, 4.2158) knots 0 0 0 1 2 2 2
  spline S486 degree 2 poles (70.8967, 4.2158) (70.9831, 4.1195) (71.1709, 4.0429) (71.2771, 4.0429) knots 0 0 0 1 2 2 2
  spline S487 degree 2 poles (71.2771, 4.0429) (71.5241, 4.0429) (71.8279, 4.3937) (71.8279, 4.7444) knots 0 0 0 1 2 2 2
  line L457 (73.258, 3.7737) -> (72.769, 3.7737)
  line L458 (72.769, 3.7737) -> (72.769, 4.3566)
  line L459 (72.769, 4.3566) -> (73.258, 4.3566)
  line L460 (73.258, 4.3566) -> (73.258, 3.7737)
  spline S488 degree 2 poles (75.77, 5.2977) (75.77, 4.4777) (75.2933, 3.7095) (74.7968, 3.7095) knots 0 0 0 1 2 2 2
  spline S489 degree 2 poles (74.7968, 3.7095) (74.293, 3.7095) (73.8212, 4.4925) (73.8212, 5.2952) knots 0 0 0 1 2 2 2
  spline S490 degree 2 poles (73.8212, 5.2952) (73.8212, 6.1202) (74.2979, 6.8835) (74.7968, 6.8835) knots 0 0 0 1 2 2 2
  spline S491 degree 2 poles (74.7968, 6.8835) (75.2983, 6.8835) (75.77, 6.0931) (75.77, 5.2977) knots 0 0 0 1 2 2 2
  spline S492 degree 2 poles (75.2464, 4.369) (75.3057, 4.5197) (75.3551, 4.984) (75.3551, 5.2977) knots 0 0 0 1 2 2 2
  spline S493 degree 2 poles (75.3551, 5.2977) (75.3551, 5.6114) (75.3057, 6.0733) (75.2439, 6.2289) knots 0 0 0 1 2 2 2
  spline S494 degree 2 poles (75.2439, 6.2289) (75.1822, 6.3845) (74.9673, 6.5451) (74.7968, 6.5451) knots 0 0 0 1 2 2 2
  spline S495 degree 2 poles (74.7968, 6.5451) (74.6264, 6.5451) (74.4066, 6.3845) (74.3424, 6.224) knots 0 0 0 1 2 2 2
  spline S496 degree 2 poles (74.3424, 6.224) (74.2806, 6.0684) (74.2361, 5.5941) (74.2361, 5.2952) knots 0 0 0 1 2 2 2
  spline S497 degree 2 poles (74.2361, 5.2952) (74.2361, 4.9741) (74.2757, 4.5444) (74.3399, 4.3764) knots 0 0 0 1 2 2 2
  spline S498 degree 2 poles (74.3399, 4.3764) (74.3992, 4.2183) (74.619, 4.0479) (74.7968, 4.0479) knots 0 0 0 1 2 2 2
  spline S499 degree 2 poles (74.7968, 4.0479) (74.9648, 4.0479) (75.1846, 4.2084) (75.2464, 4.369) knots 0 0 0 1 2 2 2
  spline S500 degree 2 poles (78.0573, 5.2977) (78.0573, 4.4777) (77.5805, 3.7095) (77.0841, 3.7095) knots 0 0 0 1 2 2 2
  spline S501 degree 2 poles (77.0841, 3.7095) (76.5802, 3.7095) (76.1084, 4.4925) (76.1084, 5.2952) knots 0 0 0 1 2 2 2
  spline S502 degree 2 poles (76.1084, 5.2952) (76.1084, 6.1202) (76.5851, 6.8835) (77.0841, 6.8835) knots 0 0 0 1 2 2 2
  spline S503 degree 2 poles (77.0841, 6.8835) (77.5855, 6.8835) (78.0573, 6.0931) (78.0573, 5.2977) knots 0 0 0 1 2 2 2
  spline S504 degree 2 poles (77.5336, 4.369) (77.5929, 4.5197) (77.6423, 4.984) (77.6423, 5.2977) knots 0 0 0 1 2 2 2
  spline S505 degree 2 poles (77.6423, 5.2977) (77.6423, 5.6114) (77.5929, 6.0733) (77.5311, 6.2289) knots 0 0 0 1 2 2 2
  spline S506 degree 2 poles (77.5311, 6.2289) (77.4694, 6.3845) (77.2545, 6.5451) (77.0841, 6.5451) knots 0 0 0 1 2 2 2
  spline S507 degree 2 poles (77.0841, 6.5451) (76.9136, 6.5451) (76.6938, 6.3845) (76.6296, 6.224) knots 0 0 0 1 2 2 2
  spline S508 degree 2 poles (76.6296, 6.224) (76.5678, 6.0684) (76.5234, 5.5941) (76.5234, 5.2952) knots 0 0 0 1 2 2 2
  spline S509 degree 2 poles (76.5234, 5.2952) (76.5234, 4.9741) (76.5629, 4.5444) (76.6271, 4.3764) knots 0 0 0 1 2 2 2
  spline S510 degree 2 poles (76.6271, 4.3764) (76.6864, 4.2183) (76.9062, 4.0479) (77.0841, 4.0479) knots 0 0 0 1 2 2 2
  spline S511 degree 2 poles (77.0841, 4.0479) (77.252, 4.0479) (77.4719, 4.2084) (77.5336, 4.369) knots 0 0 0 1 2 2 2
  spline S512 degree 2 poles (80.3445, 5.2977) (80.3445, 4.4777) (79.8678, 3.7095) (79.3713, 3.7095) knots 0 0 0 1 2 2 2
  spline S513 degree 2 poles (79.3713, 3.7095) (78.8674, 3.7095) (78.3957, 4.4925) (78.3957, 5.2952) knots 0 0 0 1 2 2 2
  spline S514 degree 2 poles (78.3957, 5.2952) (78.3957, 6.1202) (78.8724, 6.8835) (79.3713, 6.8835) knots 0 0 0 1 2 2 2
  spline S515 degree 2 poles (79.3713, 6.8835) (79.8727, 6.8835) (80.3445, 6.0931) (80.3445, 5.2977) knots 0 0 0 1 2 2 2
  spline S516 degree 2 poles (79.8208, 4.369) (79.8801, 4.5197) (79.9295, 4.984) (79.9295, 5.2977) knots 0 0 0 1 2 2 2
  spline S517 degree 2 poles (79.9295, 5.2977) (79.9295, 5.6114) (79.8801, 6.0733) (79.8184, 6.2289) knots 0 0 0 1 2 2 2
  spline S518 degree 2 poles (79.8184, 6.2289) (79.7566, 6.3845) (79.5417, 6.5451) (79.3713, 6.5451) knots 0 0 0 1 2 2 2
  spline S519 degree 2 poles (79.3713, 6.5451) (79.2009, 6.5451) (78.981, 6.3845) (78.9168, 6.224) knots 0 0 0 1 2 2 2
  spline S520 degree 2 poles (78.9168, 6.224) (78.8551, 6.0684) (78.8106, 5.5941) (78.8106, 5.2952) knots 0 0 0 1 2 2 2
  spline S521 degree 2 poles (78.8106, 5.2952) (78.8106, 4.9741) (78.8501, 4.5444) (78.9144, 4.3764) knots 0 0 0 1 2 2 2
  spline S522 degree 2 poles (78.9144, 4.3764) (78.9736, 4.2183) (79.1935, 4.0479) (79.3713, 4.0479) knots 0 0 0 1 2 2 2
  spline S523 degree 2 poles (79.3713, 4.0479) (79.5393, 4.0479) (79.7591, 4.2084) (79.8208, 4.369) knots 0 0 0 1 2 2 2
  spline S524 degree 2 poles (104.4762, 9.6069) (104.4762, 9.5138) (104.4433, 9.2921) knots 0 0 0 1 1 1
  spline S525 degree 2 poles (104.4433, 9.2921) (104.4132, 9.0951) (104.2353, 9.0951) knots 0 0 0 1 1 1
  spline S526 degree 2 poles (104.2353, 9.0951) (104.1258, 9.0951) (103.9753, 9.2374) knots 0 0 0 1 1 1
  spline S527 degree 2 poles (103.9753, 9.2374) (103.1788, 9.9928) (102.1442, 11.4188) knots 0 0 0 1 1 1
  line L461 (102.1442, 11.4188) -> (102.1332, 10.9727)
  line L462 (102.1332, 10.9727) -> (102.1278, 10.5238)
  spline S528 degree 2 poles (102.1278, 10.5238) (102.1278, 10.3623) (102.1414, 9.7082) (102.1414, 9.5439) knots 0 0 0 1 2 2 2
  spline S529 degree 2 poles (102.1414, 9.5439) (102.1414, 9.0157) (101.9362, 9.0157) knots 0 0 0 1 1 1
  spline S530 degree 2 poles (101.9362, 9.0157) (101.8294, 9.0157) (101.7665, 9.0841) knots 0 0 0 1 1 1
  spline S531 degree 2 poles (101.7665, 9.0841) (101.709, 9.1443) (101.709, 9.2292) knots 0 0 0 1 1 1
  spline S532 degree 2 poles (101.709, 9.2292) (101.709, 9.3113) (101.7336, 9.6452) (101.7336, 9.7301) knots 0 0 0 1 2 2 2
  spline S533 degree 2 poles (101.7336, 9.7301) (101.7336, 9.8505) (101.75, 10.3349) (101.75, 10.4581) knots 0 0 0 1 2 2 2
  spline S534 degree 2 poles (101.75, 10.4581) (101.75, 10.5868) (101.7391, 11.1123) (101.7391, 11.2409) knots 0 0 0 1 2 2 2
  spline S535 degree 2 poles (101.7391, 11.2409) (101.7391, 11.3641) (101.6898, 11.854) (101.6898, 11.9772) knots 0 0 0 1 2 2 2
  spline S536 degree 2 poles (101.6898, 11.9772) (101.6898, 12.0675) (101.8458, 12.218) (101.9444, 12.218) knots 0 0 0 1 2 2 2
  spline S537 degree 2 poles (101.9444, 12.218) (102.0484, 12.218) (102.2017, 11.9909) knots 0 0 0 1 1 1
  spline S538 degree 2 poles (102.2017, 11.9909) (102.6916, 11.2573) (103.0803, 10.7729) knots 0 0 0 1 1 1
  spline S539 degree 2 poles (103.0803, 10.7729) (103.5456, 10.1981) (104.1012, 9.6726) knots 0 0 0 1 1 1
  spline S540 degree 2 poles (104.1012, 9.6726) (104.1067, 9.7574) (104.1012, 9.9216) knots 0 0 0 1 1 1
  line L463 (104.1012, 9.9216) -> (104.0957, 10.168)
  spline S541 degree 2 poles (104.0957, 10.168) (104.0957, 11.0302) (104.03, 11.542) knots 0 0 0 1 1 1
  spline S542 degree 2 poles (104.03, 11.542) (104.0218, 11.5913) (103.9753, 11.7473) knots 0 0 0 1 1 1
  spline S543 degree 2 poles (103.9753, 11.7473) (103.937, 11.8814) (103.937, 11.9553) knots 0 0 0 1 1 1
  spline S544 degree 2 poles (103.937, 11.9553) (103.937, 12.1825) (104.145, 12.1825) knots 0 0 0 1 1 1
  spline S545 degree 2 poles (104.145, 12.1825) (104.4871, 12.1825) (104.4871, 10.9097) knots 0 0 0 1 1 1
  spline S546 degree 2 poles (104.4871, 10.9097) (104.4871, 10.6908) (104.4762, 9.8259) (104.4762, 9.6069) knots 0 0 0 1 2 2 2
  spline S547 degree 2 poles (106.5317, 11.6186) (106.4058, 11.6186) (106.2169, 11.6433) knots 0 0 0 1 1 1
  line L464 (106.2169, 11.6433) -> (105.8994, 11.6843)
  spline S548 degree 2 poles (105.8994, 11.6843) (105.8556, 11.1123) (105.8556, 10.595) knots 0 0 0 1 1 1
  spline S549 degree 2 poles (105.8556, 10.595) (105.8556, 10.4554) (105.8721, 10.053) (105.8721, 9.9162) knots 0 0 0 1 2 2 2
  spline S550 degree 2 poles (105.8721, 9.9162) (105.8721, 9.7301) (105.8584, 9.5795) knots 0 0 0 1 1 1
  line L465 (105.8584, 9.5795) -> (106.477, 9.5877)
  spline S551 degree 2 poles (106.477, 9.5877) (106.5591, 9.5877) (106.6713, 9.47) (106.6713, 9.3852) knots 0 0 0 1 2 2 2
  spline S552 degree 2 poles (106.6713, 9.3852) (106.6713, 9.3003) (106.5591, 9.1826) (106.477, 9.1826) knots 0 0 0 1 2 2 2
  spline S553 degree 2 poles (106.477, 9.1826) (106.3675, 9.1826) (105.9268, 9.1744) (105.8173, 9.1744) knots 0 0 0 1 2 2 2
  spline S554 degree 2 poles (105.8173, 9.1744) (105.6887, 9.1744) (105.1714, 9.1033) (105.04, 9.1033) knots 0 0 0 1 2 2 2
  spline S555 degree 2 poles (105.04, 9.1033) (104.9579, 9.1033) (104.8457, 9.2182) (104.8457, 9.3031) knots 0 0 0 1 2 2 2
  spline S556 degree 2 poles (104.8457, 9.3031) (104.8457, 9.3879) (104.9579, 9.5056) (105.04, 9.5056) knots 0 0 0 1 2 2 2
  spline S557 degree 2 poles (105.04, 9.5056) (105.1686, 9.5056) (105.4615, 9.5467) knots 0 0 0 1 1 1
  spline S558 degree 2 poles (105.4615, 9.5467) (105.4807, 9.7054) (105.4807, 9.9107) knots 0 0 0 1 1 1
  spline S559 degree 2 poles (105.4807, 9.9107) (105.4807, 10.0448) (105.456, 10.4362) (105.456, 10.5676) knots 0 0 0 1 2 2 2
  spline S560 degree 2 poles (105.456, 10.5676) (105.456, 11.0219) (105.5108, 11.7007) knots 0 0 0 1 1 1
  line L466 (105.5108, 11.7007) -> (105.2562, 11.6925)
  line L467 (105.2562, 11.6925) -> (104.9989, 11.6871)
  spline S561 degree 2 poles (104.9989, 11.6871) (104.9168, 11.6871) (104.8019, 11.802) (104.8019, 11.8896) knots 0 0 0 1 2 2 2
  spline S562 degree 2 poles (104.8019, 11.8896) (104.8019, 12.073) (104.9853, 12.0894) knots 0 0 0 1 1 1
  spline S563 degree 2 poles (104.9853, 12.0894) (105.144, 12.1058) (105.5819, 12.1058) knots 0 0 0 1 1 1
  spline S564 degree 2 poles (105.5819, 12.1058) (105.9706, 12.1058) (106.5591, 12.021) knots 0 0 0 1 1 1
  spline S565 degree 2 poles (106.5591, 12.021) (106.7342, 11.9963) (106.7342, 11.8102) knots 0 0 0 1 1 1
  spline S566 degree 2 poles (106.7342, 11.8102) (106.7342, 11.7172) (106.6686, 11.6624) knots 0 0 0 1 1 1
  spline S567 degree 2 poles (106.6686, 11.6624) (106.6083, 11.6186) (106.5317, 11.6186) knots 0 0 0 1 1 1
  spline S568 degree 2 poles (107.1174, 9.6589) (107.1147, 9.741) (107.2324, 9.845) (107.3145, 9.845) knots 0 0 0 1 2 2 2
  spline S569 degree 2 poles (107.3145, 9.845) (107.4103, 9.845) (107.4842, 9.7355) knots 0 0 0 1 1 1
  spline S570 degree 2 poles (107.4842, 9.7355) (107.5855, 9.585) (107.6621, 9.533) knots 0 0 0 1 1 1
  spline S571 degree 2 poles (107.6621, 9.533) (107.8291, 9.4235) (108.1466, 9.4235) knots 0 0 0 1 1 1
  spline S572 degree 2 poles (108.1466, 9.4235) (108.4531, 9.4235) (108.7131, 9.5549) knots 0 0 0 1 1 1
  spline S573 degree 2 poles (108.7131, 9.5549) (109.0471, 9.7246) (109.0471, 10.0229) knots 0 0 0 1 1 1
  spline S574 degree 2 poles (109.0471, 10.0229) (109.0471, 10.272) (108.7652, 10.4143) knots 0 0 0 1 1 1
  spline S575 degree 2 poles (108.7652, 10.4143) (108.5298, 10.5375) (108.1794, 10.5484) knots 0 0 0 1 1 1
  spline S576 degree 2 poles (108.1794, 10.5484) (107.8701, 10.5594) (107.6512, 10.6853) knots 0 0 0 1 1 1
  spline S577 degree 2 poles (107.6512, 10.6853) (107.372, 10.844) (107.372, 11.1396) knots 0 0 0 1 1 1
  spline S578 degree 2 poles (107.372, 11.1396) (107.372, 11.49) (107.7689, 11.7774) knots 0 0 0 1 1 1
  spline S579 degree 2 poles (107.7689, 11.7774) (108.1466, 12.0511) (108.5517, 12.0511) knots 0 0 0 1 1 1
  spline S580 degree 2 poles (108.5517, 12.0511) (108.7405, 12.0511) (108.9814, 11.9854) knots 0 0 0 1 1 1
  spline S581 degree 2 poles (108.9814, 11.9854) (109.2989, 11.9005) (109.2989, 11.7692) knots 0 0 0 1 1 1
  spline S582 degree 2 poles (109.2989, 11.7692) (109.2989, 11.5967) (109.1237, 11.5967) knots 0 0 0 1 1 1
  spline S583 degree 2 poles (109.1237, 11.5967) (109.0443, 11.5967) (108.6529, 11.6816) (108.5434, 11.6788) knots 0 0 0 1 2 2 2
  spline S584 degree 2 poles (108.5434, 11.6788) (108.2369, 11.6761) (108.0234, 11.5283) knots 0 0 0 1 1 1
  spline S585 degree 2 poles (108.0234, 11.5283) (107.8044, 11.3778) (107.8044, 11.1615) knots 0 0 0 1 1 1
  spline S586 degree 2 poles (107.8044, 11.1615) (107.8044, 11.0001) (108.0946, 10.9316) knots 0 0 0 1 1 1
  spline S587 degree 2 poles (108.0946, 10.9316) (108.2041, 10.907) (108.5133, 10.8851) knots 0 0 0 1 1 1
  spline S588 degree 2 poles (108.5133, 10.8851) (108.9622, 10.8523) (109.214, 10.6032) knots 0 0 0 1 1 1
  spline S589 degree 2 poles (109.214, 10.6032) (109.4467, 10.376) (109.4467, 10.0476) knots 0 0 0 1 1 1
  spline S590 degree 2 poles (109.4467, 10.0476) (109.4467, 9.5795) (109.0142, 9.3003) knots 0 0 0 1 1 1
  spline S591 degree 2 poles (109.0142, 9.3003) (108.6392, 9.0595) (108.1466, 9.0595) knots 0 0 0 1 1 1
  spline S592 degree 2 poles (108.1466, 9.0595) (107.7853, 9.0595) (107.4897, 9.1963) knots 0 0 0 1 1 1
  spline S593 degree 2 poles (107.4897, 9.1963) (107.1229, 9.366) (107.1174, 9.6589) knots 0 0 0 1 1 1
  spline S594 degree 2 poles (112.3151, 11.6515) (112.1701, 11.6515) (111.8662, 11.6761) knots 0 0 0 1 1 1
  spline S595 degree 2 poles (111.8662, 11.6761) (111.5734, 11.698) (111.4201, 11.6953) knots 0 0 0 1 1 1
  line L468 (111.4201, 11.6953) -> (111.2805, 11.6953)
  spline S596 degree 2 poles (111.2805, 11.6953) (111.286, 11.4243) (111.3325, 10.8139) knots 0 0 0 1 1 1